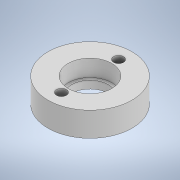
# Autodesk Inventor part: wheel_base_cover
Saved by Autodesk Inventor 2022 (Build 260153000, 153)
## iProperties
Created: 2023-03-17
Part Number: wheel_base_cover
Material: 一般
Document SubType Name: Modeling
Designer: JOU
Density: 1 g/cm^3
Appearance: 預設
Author: JOU
Autodesk Inventor part; units mm, degrees
ref_plane "YZ Plane" through (0, 0, 0) normal (1, 0, 0) x (0, 1, 0)
ref_plane "XZ Plane" through (0, 0, 0) normal (0, 1, 0) x (-1, 0, 0)
ref_plane "XY Plane" through (0, 0, 0) normal (0, 0, 1) x (1, 0, 0)
sketch "草圖1" plane through (0, 0, 0) normal (0, 1, 0) x (-1, 0, 0)
  circle A0 centre (0, 0) radius 12.5
  circle A1 centre (0, 8.5) radius 1.5
  circle A2 centre (0, -8.5) radius 1.5
  dimension "d0" = 25
  dimension "d1" = 17
  dimension "d2" = 8.5
  dimension "d3" = 3
  dimension "d4" = 3
  constraints: 3 centre point, 2 vertical alignment, 1 coincident
  measures "d0" diameter of A0
  measures "d1" distance of A2.centre A1.centre
  measures "d2" distance of point (0, 0) A2.centre
  measures "d3" diameter of A2
  measures "d4" diameter of A1
extrude "擠出1" add sketch "草圖1" along normal blind 6
sketch "草圖2" plane through (0, 6, 0) normal (0, 1, 0) x (1, 0, 0)
  circle A0 centre (0, 0) radius 5.5
  dimension "d7" = 11
  constraints: 1 centre point, 1 coincident
  measures "d7" diameter of A0
extrude "擠出2" cut sketch "草圖2" against normal through all
sketch "草圖3" plane through (0, 6, 0) normal (0, 1, 0) x (1, 0, 0)
  circle A0 centre (0, 0) radius 6.5
  dimension "d10" = 13
  constraints: 1 centre point, 1 coincident
  measures "d10" diameter of A0
extrude "擠出3" cut sketch "草圖3" against normal blind 5
move faces "移動1" translate (0, -1.25, 0) faces at (3.8939, 0, -7.6516)
